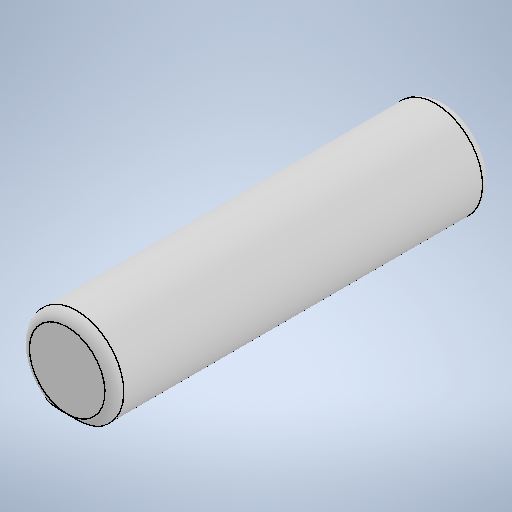
# Autodesk Inventor part: plate_joint_shaft
Saved by Autodesk Inventor 2026.3 (Build 303398000, 398)
## iProperties
Created: 2026-01-26
Part Number: plate_joint_shaft
Material: Generic
Document SubType Name: Modeling
Designer: gakut
Density: 1 g/cm^3
Appearance: Default
Author: gakut
## iProperties of the stored document plate_joint_shaft_3DPrint.ipt
Created: 2026-01-27
Part Number: plate_joint_shaft_3DPrint
Material: Generic
Document SubType Name: Modeling
Designer: gakut
Density: 1 g/cm^3
Appearance: Default
Author: gakut
Autodesk Inventor part; units mm, degrees
ref_plane "YZ Plane" through (0, 0, 0) normal (1, 0, 0) x (0, 1, 0)
ref_plane "XZ Plane" through (0, 0, 0) normal (0, 1, 0) x (-1, 0, 0)
ref_plane "XY Plane" through (0, 0, 0) normal (0, 0, 1) x (1, 0, 0)
sketch "Sketch1" plane through (0, 0, 0) normal (0, 0, 1) x (1, 0, 0)
  circle A0 centre (0, 0) radius 5
  line L0 (-3, -4) -> (3, -4)
  dimension "d3" = 10
  dimension "d4" = 1
  constraints: 2 coincident, 2 end point, 2 point on circle, 1 centre point, 1 horizontal
  measures "d3" diameter of A0
  measures "d4" distance edge to line of A0 L0
extrude "Extrusion1" add sketch "Sketch1" along normal mid plane 40 contours A0 L0 picked at (0.9594, -1.3039)
fillet "Fillet1" radius 1 2 edges at (0, 5, 20) (0, 5, -20)
body "Solid1"
